Autodesk Inventor part; units mm, degrees
(part 6 of 6)
  arc A193 (71.9714, -302.9558) -> (71.5938, -302.4165) centre (71.5537, -302.8464) ccw
  arc A194 (71.5938, -302.4165) -> (70.7191, -302.3472) centre (68.6893, -333.536) ccw
  arc A195 (70.7191, -302.3472) -> (70.2313, -302.8189) centre (70.6894, -302.8046) ccw
  arc A196 (68.6893, -304.4648) -> (70.2313, -302.8189) centre (68.6351, -302.8687) ccw
  arc A197 (67.1472, -302.8189) -> (68.6893, -304.4648) centre (68.6385, -302.9671) ccw
  arc A198 (67.1472, -302.8189) -> (66.6899, -302.3453) centre (66.7175, -302.7762) ccw
  arc A199 (66.6899, -302.3453) -> (65.8152, -302.4137) centre (68.6893, -333.536) ccw
  circle A200 centre (68.6893, -333.536) radius 14.1111
  circle A201 centre (73.3883, -316.503) radius 2.0193
  circle A202 centre (51.5888, -337.983) radius 2.0193
  circle A203 centre (85.7897, -329.089) radius 2.0193
  circle A204 centre (56.2878, -320.95) radius 2.0193
  circle A205 centre (63.9903, -350.5689) radius 2.0193
  circle A206 centre (81.0907, -346.1219) radius 2.0193
  line L0 (-99.6407, 85.3463) -> (-99.6407, -123.6777) projected
  line L1 (-99.6407, -123.6777) -> (-99.6407, -461.902)
  arc A207 (-67.782, -300.7465) -> (-68.1901, -301.2886) centre (-67.7399, -301.2029) ccw
  arc A208 (-69.4556, -303.1555) -> (-68.1901, -301.2886) centre (-69.7588, -301.5876) ccw
  arc A209 (-71.2362, -301.7711) -> (-69.4556, -303.1555) centre (-69.7401, -301.6842) ccw
  arc A210 (-71.2362, -301.7711) -> (-71.762, -301.3749) centre (-71.6673, -301.7962) ccw
  arc A211 (-71.762, -301.3749) -> (-72.6152, -301.5793) centre (-64.9079, -331.8688) ccw
  arc A212 (-72.6152, -301.5793) -> (-72.9334, -302.1786) centre (-72.5022, -302.0234) ccw
  arc A213 (-73.8914, -304.2205) -> (-72.9334, -302.1786) centre (-74.4361, -302.7192) ccw
  arc A214 (-75.8666, -303.1316) -> (-73.8914, -304.2205) centre (-74.4025, -302.8117) ccw
  arc A215 (-75.8666, -303.1316) -> (-76.4479, -302.8225) centre (-76.2884, -303.2238) ccw
  arc A216 (-76.4479, -302.8225) -> (-77.2586, -303.1579) centre (-64.9079, -331.8688) ccw
  arc A217 (-77.2586, -303.1579) -> (-77.4792, -303.7996) centre (-77.0775, -303.5789) ccw
  arc A218 (-78.1059, -305.9662) -> (-77.4792, -303.7996) centre (-78.8788, -304.5687) ccw
  arc A219 (-80.2272, -305.1997) -> (-78.1059, -305.9662) centre (-78.8312, -304.6547) ccw
  arc A220 (-80.2272, -305.1997) -> (-80.8496, -304.9854) centre (-80.6294, -305.3568) ccw
  arc A221 (-80.8496, -304.9854) -> (-81.598, -305.4434) centre (-64.9079, -331.8688) ccw
  arc A222 (-81.598, -305.4434) -> (-81.7154, -306.1117) centre (-81.3532, -305.8309) ccw
  arc A223 (-81.9955, -308.3497) -> (-81.7154, -306.1117) centre (-82.9774, -307.0903) ccw
  arc A224 (-84.2105, -307.9245) -> (-81.9955, -308.3497) centre (-82.917, -307.1679) ccw
  arc A225 (-84.2105, -307.9245) -> (-84.8589, -307.8102) centre (-84.5832, -308.1426) ccw
  arc A226 (-84.8589, -307.8102) -> (-85.5263, -308.3797) centre (-64.9079, -331.8688) ccw
  arc A227 (-85.5263, -308.3797) -> (-85.5378, -309.0581) centre (-85.224, -308.7241) ccw
  arc A228 (-85.4643, -311.3124) -> (-85.5378, -309.0581) centre (-86.6312, -310.2221) ccw
  arc A229 (-87.7186, -311.2389) -> (-85.4643, -311.3124) centre (-86.5593, -310.2892) ccw
  arc A230 (-87.7186, -311.2389) -> (-88.3768, -311.2274) centre (-88.0526, -311.5126) ccw
  arc A231 (-88.3768, -311.2274) -> (-88.947, -311.8943) centre (-64.9079, -331.8688) ccw
  arc A232 (-88.947, -311.8943) -> (-88.8522, -312.5662) centre (-88.5945, -312.1872) ccw
  arc A233 (-88.427, -314.7812) -> (-88.8522, -312.5662) centre (-89.75, -313.8868) ccw
  arc A234 (-90.6649, -315.0613) -> (-88.427, -314.7812) centre (-89.6685, -313.9419) ccw
  arc A235 (-90.6649, -315.0613) -> (-91.3169, -315.1529) centre (-90.9521, -315.3838) ccw
  arc A236 (-91.3169, -315.1529) -> (-91.7757, -315.9007) centre (-64.9079, -331.8688) ccw
  arc A237 (-91.7757, -315.9007) -> (-91.577, -316.5495) centre (-91.3817, -316.1349) ccw
  arc A238 (-90.8105, -318.6707) -> (-91.577, -316.5495) centre (-92.2572, -317.9944) ccw
  arc A239 (-92.9771, -319.2975) -> (-90.8105, -318.6707) centre (-92.1681, -318.036) ccw
  arc A240 (-92.9771, -319.2975) -> (-93.6067, -319.4899) centre (-93.2102, -319.661) ccw
  arc A241 (-93.6067, -319.4899) -> (-93.9429, -320.3004) centre (-64.9079, -331.8688) ccw
  arc A242 (-93.9429, -320.3004) -> (-93.6451, -320.9101) centre (-93.5171, -320.47) ccw
  arc A243 (-92.5562, -322.8853) -> (-93.6451, -320.9101) centre (-94.0909, -322.4436) ccw
  arc A244 (-94.5981, -323.8433) -> (-92.5562, -322.8853) centre (-93.9964, -322.4708) ccw
  arc A245 (-94.5981, -323.8433) -> (-95.1899, -324.1318) centre (-94.7715, -324.2387) ccw
  arc A246 (-95.1899, -324.1318) -> (-95.3951, -324.9849) centre (-64.9079, -331.8688) ccw
  arc A247 (-95.3951, -324.9849) -> (-95.0056, -325.5405) centre (-94.9481, -325.0858) ccw
  arc A248 (-93.6212, -327.321) -> (-95.0056, -325.5405) centre (-95.206, -327.1248) ccw
  arc A249 (-95.488, -328.5866) -> (-93.6212, -327.321) centre (-95.1084, -327.1369) ccw
  arc A250 (-95.488, -328.5866) -> (-96.0274, -328.9642) centre (-95.5974, -329.0043) ccw
  arc A251 (-96.0274, -328.9642) -> (-96.0966, -329.8389) centre (-64.9079, -331.8688) ccw
  arc A252 (-96.0966, -329.8389) -> (-95.625, -330.3267) centre (-95.6393, -329.8686) ccw
  arc A253 (-93.9791, -331.8688) -> (-95.625, -330.3267) centre (-95.5751, -331.9229) ccw
  arc A254 (-95.625, -333.4108) -> (-93.9791, -331.8688) centre (-95.4768, -331.9196) ccw
  arc A255 (-95.625, -333.4108) -> (-96.0986, -333.8681) centre (-95.6677, -333.8405) ccw
  arc A256 (-96.0986, -333.8681) -> (-96.0302, -334.7429) centre (-64.9079, -331.8688) ccw
  arc A257 (-96.0302, -334.7429) -> (-95.488, -335.1509) centre (-95.5738, -334.7007) ccw
  arc A258 (-93.6212, -336.4165) -> (-95.488, -335.1509) centre (-95.1891, -336.7196) ccw
  arc A259 (-95.0056, -338.1971) -> (-93.6212, -336.4165) centre (-95.0925, -336.701) ccw
  arc A260 (-95.0056, -338.1971) -> (-95.4018, -338.7228) centre (-94.9805, -338.6281) ccw
  arc A261 (-95.4018, -338.7228) -> (-95.1974, -339.5761) centre (-64.9079, -331.8688) ccw
  arc A262 (-95.1974, -339.5761) -> (-94.5981, -339.8943) centre (-94.7533, -339.4631) ccw
  arc A263 (-92.5562, -340.8523) -> (-94.5981, -339.8943) centre (-94.0574, -341.3969) ccw
  arc A264 (-93.6451, -342.8275) -> (-92.5562, -340.8523) centre (-93.965, -341.3634) ccw
  arc A265 (-93.6451, -342.8275) -> (-93.9542, -343.4087) centre (-93.5529, -343.2493) ccw
  arc A266 (-93.9542, -343.4087) -> (-93.6188, -344.2195) centre (-64.9079, -331.8688) ccw
  arc A267 (-93.6188, -344.2195) -> (-92.9771, -344.44) centre (-93.1978, -344.0384) ccw
  arc A268 (-90.8105, -345.0668) -> (-92.9771, -344.44) centre (-92.208, -345.8396) ccw
  arc A269 (-91.577, -347.188) -> (-90.8105, -345.0668) centre (-92.1219, -345.792) ccw
  arc A270 (-91.577, -347.188) -> (-91.7913, -347.8105) centre (-91.4199, -347.5902) ccw
  arc A271 (-91.7913, -347.8105) -> (-91.3333, -348.5588) centre (-64.9079, -331.8688) ccw
  arc A272 (-91.3333, -348.5588) -> (-90.6649, -348.6763) centre (-90.9458, -348.3141) ccw
  arc A273 (-88.427, -348.9564) -> (-90.6649, -348.6763) centre (-89.6864, -349.9383) ccw
  arc A274 (-88.8522, -351.1714) -> (-88.427, -348.9564) centre (-89.6088, -349.8778) ccw
  arc A275 (-88.8522, -351.1714) -> (-88.9665, -351.8197) centre (-88.6341, -351.5441) ccw
  arc A276 (-88.9665, -351.8197) -> (-88.397, -352.4872) centre (-64.9079, -331.8688) ccw
  arc A277 (-88.397, -352.4872) -> (-87.7186, -352.4986) centre (-88.0526, -352.1848) ccw
  arc A278 (-85.4643, -352.4252) -> (-87.7186, -352.4986) centre (-86.5546, -353.592) ccw
  arc A279 (-85.5378, -354.6794) -> (-85.4643, -352.4252) centre (-86.4875, -353.5202) ccw
  arc A280 (-85.5378, -354.6794) -> (-85.5493, -355.3377) centre (-85.2641, -355.0134) ccw
  arc A281 (-85.5493, -355.3377) -> (-84.8824, -355.9078) centre (-64.9079, -331.8688) ccw
  arc A282 (-84.8824, -355.9078) -> (-84.2105, -355.813) centre (-84.5895, -355.5553) ccw
  arc A283 (-81.9955, -355.3878) -> (-84.2105, -355.813) centre (-82.8899, -356.7109) ccw
  arc A284 (-81.7154, -357.6258) -> (-81.9955, -355.3878) centre (-82.8348, -356.6294) ccw
  arc A285 (-81.7154, -357.6258) -> (-81.6238, -358.2778) centre (-81.3929, -357.9129) ccw
  arc A286 (-81.6238, -358.2778) -> (-80.8759, -358.7366) centre (-64.9079, -331.8688) ccw
  arc A287 (-80.8759, -358.7366) -> (-80.2272, -358.5378) centre (-80.6418, -358.3426) ccw
  arc A288 (-78.1059, -357.7714) -> (-80.2272, -358.5378) centre (-78.7823, -359.218) ccw
  arc A289 (-77.4792, -359.938) -> (-78.1059, -357.7714) centre (-78.7406, -359.1289) ccw
  arc A290 (-77.4792, -359.938) -> (-77.2867, -360.5676) centre (-77.1157, -360.1711) ccw
  arc A291 (-77.2867, -360.5676) -> (-76.4763, -360.9037) centre (-64.9079, -331.8688) ccw
  arc A292 (-76.4763, -360.9037) -> (-75.8666, -360.6059) centre (-76.3067, -360.478) ccw
  arc A293 (-73.8914, -359.5171) -> (-75.8666, -360.6059) centre (-74.3331, -361.0518) ccw
  arc A294 (-72.9334, -361.559) -> (-73.8914, -359.5171) centre (-74.3059, -360.9572) ccw
  arc A295 (-72.9334, -361.559) -> (-72.6449, -362.1507) centre (-72.538, -361.7324) ccw
  arc A296 (-72.6449, -362.1507) -> (-71.7918, -362.356) centre (-64.9079, -331.8688) ccw
  arc A297 (-71.7918, -362.356) -> (-71.2362, -361.9664) centre (-71.6909, -361.9089) ccw
  arc A298 (-69.4556, -360.582) -> (-71.2362, -361.9664) centre (-69.6519, -362.1669) ccw
  arc A299 (-68.1901, -362.4489) -> (-69.4556, -360.582) centre (-69.6398, -362.0693) ccw
  arc A300 (-68.1901, -362.4489) -> (-67.8125, -362.9882) centre (-67.7723, -362.5583) ccw
  arc A301 (-67.8125, -362.9882) -> (-66.9378, -363.0575) centre (-64.9079, -331.8688) ccw
  arc A302 (-66.9378, -363.0575) -> (-66.45, -362.5858) centre (-66.908, -362.6002) ccw
  arc A303 (-64.9079, -360.9399) -> (-66.45, -362.5858) centre (-64.8538, -362.536) ccw
  arc A304 (-63.3659, -362.5858) -> (-64.9079, -360.9399) centre (-64.8571, -362.4377) ccw
  arc A305 (-63.3659, -362.5858) -> (-62.9086, -363.0595) centre (-62.9362, -362.6285) ccw
  arc A306 (-62.9086, -363.0595) -> (-62.0338, -362.991) centre (-64.9079, -331.8688) ccw
  arc A307 (-62.0338, -362.991) -> (-61.6258, -362.4489) centre (-62.076, -362.5347) ccw
  arc A308 (-60.3602, -360.582) -> (-61.6258, -362.4489) centre (-60.057, -362.15) ccw
  arc A309 (-58.5796, -361.9664) -> (-60.3602, -360.582) centre (-60.0757, -362.0534) ccw
  arc A310 (-58.5796, -361.9664) -> (-58.0539, -362.3627) centre (-58.1486, -361.9414) ccw
  arc A311 (-58.0539, -362.3627) -> (-57.2006, -362.1583) centre (-64.9079, -331.8688) ccw
  arc A312 (-57.2006, -362.1583) -> (-56.8824, -361.559) centre (-57.3136, -361.7141) ccw
  arc A313 (-55.9244, -359.5171) -> (-56.8824, -361.559) centre (-55.3797, -361.0183) ccw
  arc A314 (-53.9492, -360.6059) -> (-55.9244, -359.5171) centre (-55.4133, -360.9258) ccw
  arc A315 (-53.9492, -360.6059) -> (-53.368, -360.915) centre (-53.5274, -360.5137) ccw
  arc A316 (-53.368, -360.915) -> (-52.5572, -360.5797) centre (-64.9079, -331.8688) ccw
  arc A317 (-52.5572, -360.5797) -> (-52.3366, -359.938) centre (-52.7383, -360.1587) ccw
  arc A318 (-51.7099, -357.7714) -> (-52.3366, -359.938) centre (-50.9371, -359.1689) ccw
  arc A319 (-49.5887, -358.5378) -> (-51.7099, -357.7714) centre (-50.9847, -359.0828) ccw
  arc A320 (-49.5887, -358.5378) -> (-48.9662, -358.7522) centre (-49.1864, -358.3808) ccw
  arc A321 (-48.9662, -358.7522) -> (-48.2179, -358.2941) centre (-64.9079, -331.8688) ccw
  arc A322 (-48.2179, -358.2941) -> (-48.1004, -357.6258) centre (-48.4626, -357.9066) ccw
  arc A323 (-47.8203, -355.3878) -> (-48.1004, -357.6258) centre (-46.8384, -356.6472) ccw
  arc A324 (-45.6053, -355.813) -> (-47.8203, -355.3878) centre (-46.8989, -356.5697) ccw
  arc A325 (-45.6053, -355.813) -> (-44.957, -355.9274) centre (-45.2326, -355.595) ccw
  arc A326 (-44.957, -355.9274) -> (-44.2895, -355.3579) centre (-64.9079, -331.8688) ccw
  arc A327 (-44.2895, -355.3579) -> (-44.2781, -354.6794) centre (-44.5919, -355.0134) ccw
  arc A328 (-44.3515, -352.4252) -> (-44.2781, -354.6794) centre (-43.1846, -353.5155) ccw
  arc A329 (-42.0973, -352.4986) -> (-44.3515, -352.4252) centre (-43.2565, -353.4483) ccw
  arc A330 (-42.0973, -352.4986) -> (-41.439, -352.5102) centre (-41.7632, -352.225) ccw
  arc A331 (-41.439, -352.5102) -> (-40.8689, -351.8433) centre (-64.9079, -331.8688) ccw
  arc A332 (-40.8689, -351.8433) -> (-40.9637, -351.1714) centre (-41.2214, -351.5504) ccw
  arc A333 (-41.3889, -348.9564) -> (-40.9637, -351.1714) centre (-40.0658, -349.8507) ccw
  arc A334 (-39.1509, -348.6763) -> (-41.3889, -348.9564) centre (-40.1473, -349.7956) ccw
  arc A335 (-39.1509, -348.6763) -> (-38.4989, -348.5847) centre (-38.8638, -348.3537) ccw
  arc A336 (-38.4989, -348.5847) -> (-38.0401, -347.8368) centre (-64.9079, -331.8688) ccw
  arc A337 (-38.0401, -347.8368) -> (-38.2389, -347.188) centre (-38.4341, -347.6027) ccw
  arc A338 (-39.0053, -345.0668) -> (-38.2389, -347.188) centre (-37.5587, -345.7432) ccw
  arc A339 (-36.8387, -344.44) -> (-39.0053, -345.0668) centre (-37.6478, -345.7015) ccw
  arc A340 (-36.8387, -344.44) -> (-36.2091, -344.2476) centre (-36.6056, -344.0766) ccw
  arc A341 (-36.2091, -344.2476) -> (-35.873, -343.4372) centre (-64.9079, -331.8688) ccw
  arc A342 (-35.873, -343.4372) -> (-36.1708, -342.8275) centre (-36.2987, -343.2675) ccw
  arc A343 (-37.2596, -340.8523) -> (-36.1708, -342.8275) centre (-35.7249, -341.294) ccw
  arc A344 (-35.2177, -339.8943) -> (-37.2596, -340.8523) centre (-35.8195, -341.2668) ccw
  arc A345 (-35.2177, -339.8943) -> (-34.626, -339.6057) centre (-35.0443, -339.4988) ccw
  arc A346 (-34.626, -339.6057) -> (-34.4207, -338.7527) centre (-64.9079, -331.8688) ccw
  arc A347 (-34.4207, -338.7527) -> (-34.8103, -338.1971) centre (-34.8678, -338.6517) ccw
  arc A348 (-36.1947, -336.4165) -> (-34.8103, -338.1971) centre (-34.6098, -336.6127) ccw
  arc A349 (-34.3278, -335.1509) -> (-36.1947, -336.4165) centre (-34.7074, -336.6006) ccw
  arc A350 (-34.3278, -335.1509) -> (-33.7885, -334.7733) centre (-34.2184, -334.7332) ccw
  arc A351 (-33.7885, -334.7733) -> (-33.7192, -333.8987) centre (-64.9079, -331.8688) ccw
  arc A352 (-33.7192, -333.8987) -> (-34.1908, -333.4108) centre (-34.1765, -333.8689) ccw
  arc A353 (-35.8368, -331.8688) -> (-34.1908, -333.4108) centre (-34.2407, -331.8146) ccw
  arc A354 (-34.1908, -330.3267) -> (-35.8368, -331.8688) centre (-34.339, -331.818) ccw
  arc A355 (-34.1908, -330.3267) -> (-33.7172, -329.8694) centre (-34.1481, -329.897) ccw
  arc A356 (-33.7172, -329.8694) -> (-33.7856, -328.9947) centre (-64.9079, -331.8688) ccw
  arc A357 (-33.7856, -328.9947) -> (-34.3278, -328.5866) centre (-34.242, -329.0368) ccw
  arc A358 (-36.1947, -327.321) -> (-34.3278, -328.5866) centre (-34.6267, -327.0179) ccw
  arc A359 (-34.8103, -325.5405) -> (-36.1947, -327.321) centre (-34.7233, -327.0366) ccw
  arc A360 (-34.8103, -325.5405) -> (-34.414, -325.0147) centre (-34.8353, -325.1094) ccw
  arc A361 (-34.414, -325.0147) -> (-34.6184, -324.1615) centre (-64.9079, -331.8688) ccw
  arc A362 (-34.6184, -324.1615) -> (-35.2177, -323.8433) centre (-35.0626, -324.2745) ccw
  arc A363 (-37.2596, -322.8853) -> (-35.2177, -323.8433) centre (-35.7584, -322.3406) ccw
  arc A364 (-36.1708, -320.9101) -> (-37.2596, -322.8853) centre (-35.8509, -322.3741) ccw
  arc A365 (-36.1708, -320.9101) -> (-35.8616, -320.3288) centre (-36.2629, -320.4882) ccw
  arc A366 (-35.8616, -320.3288) -> (-36.197, -319.518) centre (-64.9079, -331.8688) ccw
  arc A367 (-36.197, -319.518) -> (-36.8387, -319.2975) centre (-36.618, -319.6991) ccw
  arc A368 (-39.0053, -318.6707) -> (-36.8387, -319.2975) centre (-37.6078, -317.8979) ccw
  arc A369 (-38.2389, -316.5495) -> (-39.0053, -318.6707) centre (-37.6939, -317.9455) ccw
  arc A370 (-38.2389, -316.5495) -> (-38.0245, -315.927) centre (-38.3959, -316.1473) ccw
  arc A371 (-38.0245, -315.927) -> (-38.4826, -315.1787) centre (-64.9079, -331.8688) ccw
  arc A372 (-38.4826, -315.1787) -> (-39.1509, -315.0613) centre (-38.8701, -315.4235) ccw
  arc A373 (-41.3889, -314.7812) -> (-39.1509, -315.0613) centre (-40.1294, -313.7992) ccw
  arc A374 (-40.9637, -312.5662) -> (-41.3889, -314.7812) centre (-40.207, -313.8597) ccw
  arc A375 (-40.9637, -312.5662) -> (-40.8493, -311.9178) centre (-41.1817, -312.1935) ccw
  arc A376 (-40.8493, -311.9178) -> (-41.4188, -311.2504) centre (-64.9079, -331.8688) ccw
  arc A377 (-41.4188, -311.2504) -> (-42.0973, -311.2389) centre (-41.7632, -311.5527) ccw
  arc A378 (-44.3515, -311.3124) -> (-42.0973, -311.2389) centre (-43.2612, -310.1455) ccw
  arc A379 (-44.2781, -309.0581) -> (-44.3515, -311.3124) centre (-43.3284, -310.2174) ccw
  arc A380 (-44.2781, -309.0581) -> (-44.2665, -308.3999) centre (-44.5517, -308.7241) ccw
  arc A381 (-44.2665, -308.3999) -> (-44.9334, -307.8297) centre (-64.9079, -331.8688) ccw
  arc A382 (-44.9334, -307.8297) -> (-45.6053, -307.9245) centre (-45.2263, -308.1822) ccw
  arc A383 (-47.8203, -308.3497) -> (-45.6053, -307.9245) centre (-46.926, -307.0267) ccw
  arc A384 (-48.1004, -306.1117) -> (-47.8203, -308.3497) centre (-46.9811, -307.1082) ccw
  arc A385 (-48.1004, -306.1117) -> (-48.192, -305.4598) centre (-48.4229, -305.8246) ccw
  arc A386 (-48.192, -305.4598) -> (-48.9399, -305.001) centre (-64.9079, -331.8688) ccw
  arc A387 (-48.9399, -305.001) -> (-49.5887, -305.1997) centre (-49.174, -305.3949) ccw
  arc A388 (-51.7099, -305.9662) -> (-49.5887, -305.1997) centre (-51.0335, -304.5195) ccw
  arc A389 (-52.3366, -303.7996) -> (-51.7099, -305.9662) centre (-51.0752, -304.6086) ccw
  arc A390 (-52.3366, -303.7996) -> (-52.5291, -303.17) centre (-52.7001, -303.5665) ccw
  arc A391 (-52.5291, -303.17) -> (-53.3395, -302.8338) centre (-64.9079, -331.8688) ccw
  arc A392 (-53.3395, -302.8338) -> (-53.9492, -303.1316) centre (-53.5092, -303.2596) ccw
  arc A393 (-55.9244, -304.2205) -> (-53.9492, -303.1316) centre (-55.4827, -302.6858) ccw
  arc A394 (-56.8824, -302.1786) -> (-55.9244, -304.2205) centre (-55.5099, -302.7803) ccw
  arc A395 (-56.8824, -302.1786) -> (-57.171, -301.5868) centre (-57.2779, -302.0052) ccw
  arc A396 (-57.171, -301.5868) -> (-58.024, -301.3816) centre (-64.9079, -331.8688) ccw
  arc A397 (-58.024, -301.3816) -> (-58.5796, -301.7711) centre (-58.125, -301.8286) ccw
  arc A398 (-60.3602, -303.1555) -> (-58.5796, -301.7711) centre (-60.164, -301.5707) ccw
  arc A399 (-61.6258, -301.2886) -> (-60.3602, -303.1555) centre (-60.1761, -301.6683) ccw
  arc A400 (-61.6258, -301.2886) -> (-62.0034, -300.7493) centre (-62.0435, -301.1793) ccw
  arc A401 (-62.0034, -300.7493) -> (-62.878, -300.6801) centre (-64.9079, -331.8688) ccw
  arc A402 (-62.878, -300.6801) -> (-63.3659, -301.1517) centre (-62.9078, -301.1374) ccw
  arc A403 (-64.9079, -302.7976) -> (-63.3659, -301.1517) centre (-64.9621, -301.2016) ccw
  arc A404 (-66.45, -301.1517) -> (-64.9079, -302.7976) centre (-64.9587, -301.2999) ccw
  arc A405 (-66.45, -301.1517) -> (-66.9073, -300.6781) centre (-66.8797, -301.109) ccw
  arc A406 (-66.9073, -300.6781) -> (-67.782, -300.7465) centre (-64.9079, -331.8688) ccw
  circle A407 centre (-64.9079, -331.8688) radius 14.1111
  circle A408 centre (-60.2089, -314.8359) radius 2.0193
  circle A409 centre (-82.0084, -336.3158) radius 2.0193
  circle A410 centre (-47.8075, -327.4218) radius 2.0193
  circle A411 centre (-77.3094, -319.2829) radius 2.0193
  circle A412 centre (-69.6069, -348.9017) radius 2.0193
  circle A413 centre (-52.5065, -344.4547) radius 2.0193
  arc A414 (-1.7986, -301.6927) -> (-2.2066, -302.2349) centre (-1.7564, -302.1491) ccw
  arc A415 (-3.4722, -304.1017) -> (-2.2066, -302.2349) centre (-3.7754, -302.5338) ccw
  arc A416 (-5.2528, -302.7173) -> (-3.4722, -304.1017) centre (-3.7567, -302.6304) ccw
  arc A417 (-5.2528, -302.7173) -> (-5.7785, -302.3211) centre (-5.6839, -302.7424) ccw
  arc A418 (-5.7785, -302.3211) -> (-6.6318, -302.5255) centre (1.0755, -332.815) ccw
  arc A419 (-6.6318, -302.5255) -> (-6.95, -303.1248) centre (-6.5188, -302.9696) ccw
  arc A420 (-7.908, -305.1667) -> (-6.95, -303.1248) centre (-8.4527, -303.6655) ccw
  arc A421 (-9.8832, -304.0778) -> (-7.908, -305.1667) centre (-8.4191, -303.7579) ccw
  arc A422 (-9.8832, -304.0778) -> (-10.4645, -303.7687) centre (-10.305, -304.17) ccw
  arc A423 (-10.4645, -303.7687) -> (-11.2752, -304.1041) centre (1.0755, -332.815) ccw
  arc A424 (-11.2752, -304.1041) -> (-11.4958, -304.7458) centre (-11.0941, -304.5251) ccw
  arc A425 (-12.1225, -306.9124) -> (-11.4958, -304.7458) centre (-12.8954, -305.5149) ccw
  arc A426 (-14.2437, -306.1459) -> (-12.1225, -306.9124) centre (-12.8478, -305.601) ccw
  arc A427 (-14.2437, -306.1459) -> (-14.8662, -305.9316) centre (-14.646, -306.303) ccw
  arc A428 (-14.8662, -305.9316) -> (-15.6145, -306.3896) centre (1.0755, -332.815) ccw
  arc A429 (-15.6145, -306.3896) -> (-15.732, -307.058) centre (-15.3698, -306.7771) ccw
  arc A430 (-16.0121, -309.2959) -> (-15.732, -307.058) centre (-16.994, -308.0365) ccw
  arc A431 (-18.2271, -308.8707) -> (-16.0121, -309.2959) centre (-16.9335, -308.1141) ccw
  arc A432 (-18.2271, -308.8707) -> (-18.8754, -308.7564) centre (-18.5998, -309.0888) ccw
  arc A433 (-18.8754, -308.7564) -> (-19.5429, -309.3259) centre (1.0755, -332.815) ccw
  arc A434 (-19.5429, -309.3259) -> (-19.5544, -310.0043) centre (-19.2406, -309.6703) ccw
  arc A435 (-19.4809, -312.2586) -> (-19.5544, -310.0043) centre (-20.6478, -311.1683) ccw
  arc A436 (-21.7351, -312.1851) -> (-19.4809, -312.2586) centre (-20.5759, -311.2354) ccw
  arc A437 (-21.7351, -312.1851) -> (-22.3934, -312.1736) centre (-22.0692, -312.4588) ccw
  arc A438 (-22.3934, -312.1736) -> (-22.9636, -312.8405) centre (1.0755, -332.815) ccw
  arc A439 (-22.9636, -312.8405) -> (-22.8687, -313.5124) centre (-22.6111, -313.1334) ccw
  arc A440 (-22.4436, -315.7274) -> (-22.8687, -313.5124) centre (-23.7666, -314.833) ccw
  arc A441 (-24.6815, -316.0075) -> (-22.4436, -315.7274) centre (-23.6851, -314.8881) ccw
  arc A442 (-24.6815, -316.0075) -> (-25.3335, -316.0991) centre (-24.9686, -316.33) ccw
  arc A443 (-25.3335, -316.0991) -> (-25.7923, -316.847) centre (1.0755, -332.815) ccw
  arc A444 (-25.7923, -316.847) -> (-25.5935, -317.4957) centre (-25.3983, -317.0811) ccw
  arc A445 (-24.8271, -319.617) -> (-25.5935, -317.4957) centre (-26.2738, -318.9406) ccw
  arc A446 (-26.9937, -320.2437) -> (-24.8271, -319.617) centre (-26.1846, -318.9823) ccw
  arc A447 (-26.9937, -320.2437) -> (-27.6233, -320.4362) centre (-27.2268, -320.6072) ccw
  arc A448 (-27.6233, -320.4362) -> (-27.9595, -321.2466) centre (1.0755, -332.815) ccw
  arc A449 (-27.9595, -321.2466) -> (-27.6616, -321.8563) centre (-27.5337, -321.4162) ccw
  arc A450 (-26.5728, -323.8315) -> (-27.6616, -321.8563) centre (-28.1075, -323.3898) ccw
  arc A451 (-28.6147, -324.7895) -> (-26.5728, -323.8315) centre (-28.0129, -323.417) ccw
  arc A452 (-28.6147, -324.7895) -> (-29.2064, -325.078) centre (-28.7881, -325.1849) ccw
  arc A453 (-29.2064, -325.078) -> (-29.4117, -325.9311) centre (1.0755, -332.815) ccw
  arc A454 (-29.4117, -325.9311) -> (-29.0222, -326.4867) centre (-28.9646, -326.032) ccw
  arc A455 (-27.6377, -328.2673) -> (-29.0222, -326.4867) centre (-29.2226, -328.071) ccw
  arc A456 (-29.5046, -329.5328) -> (-27.6377, -328.2673) centre (-29.125, -328.0831) ccw
  arc A457 (-29.5046, -329.5328) -> (-30.0439, -329.9104) centre (-29.614, -329.9506) ccw
  arc A458 (-30.0439, -329.9104) -> (-30.1132, -330.7851) centre (1.0755, -332.815) ccw
  arc A459 (-30.1132, -330.7851) -> (-29.6416, -331.2729) centre (-29.6559, -330.8149) ccw
  arc A460 (-27.9957, -332.815) -> (-29.6416, -331.2729) centre (-29.5917, -332.8691) ccw
  arc A461 (-29.6416, -334.357) -> (-27.9957, -332.815) centre (-29.4934, -332.8658) ccw
  arc A462 (-29.6416, -334.357) -> (-30.1152, -334.8143) centre (-29.6843, -334.7867) ccw
  arc A463 (-30.1152, -334.8143) -> (-30.0468, -335.6891) centre (1.0755, -332.815) ccw
  arc A464 (-30.0468, -335.6891) -> (-29.5046, -336.0971) centre (-29.5904, -335.6469) ccw
  arc A465 (-27.6377, -337.3627) -> (-29.5046, -336.0971) centre (-29.2057, -337.6659) ccw
  arc A466 (-29.0222, -339.1433) -> (-27.6377, -337.3627) centre (-29.1091, -337.6472) ccw
  arc A467 (-29.0222, -339.1433) -> (-29.4184, -339.669) centre (-28.9971, -339.5743) ccw
  arc A468 (-29.4184, -339.669) -> (-29.214, -340.5223) centre (1.0755, -332.815) ccw
  arc A469 (-29.214, -340.5223) -> (-28.6147, -340.8405) centre (-28.7699, -340.4093) ccw
  arc A470 (-26.5728, -341.7985) -> (-28.6147, -340.8405) centre (-28.074, -342.3432) ccw
  arc A471 (-27.6616, -343.7737) -> (-26.5728, -341.7985) centre (-27.9816, -342.3096) ccw
  arc A472 (-27.6616, -343.7737) -> (-27.9708, -344.3549) centre (-27.5695, -344.1955) ccw
  arc A473 (-27.9708, -344.3549) -> (-27.6354, -345.1657) centre (1.0755, -332.815) ccw
  arc A474 (-27.6354, -345.1657) -> (-26.9937, -345.3863) centre (-27.2144, -344.9846) ccw
  arc A475 (-24.8271, -346.013) -> (-26.9937, -345.3863) centre (-26.2246, -346.7858) ccw
  arc A476 (-25.5935, -348.1342) -> (-24.8271, -346.013) centre (-26.1385, -346.7382) ccw
  arc A477 (-25.5935, -348.1342) -> (-25.8079, -348.7567) centre (-25.4365, -348.5365) ccw
  arc A478 (-25.8079, -348.7567) -> (-25.3498, -349.505) centre (1.0755, -332.815) ccw
  arc A479 (-25.3498, -349.505) -> (-24.6815, -349.6225) centre (-24.9624, -349.2603) ccw
  arc A480 (-22.4436, -349.9026) -> (-24.6815, -349.6225) centre (-23.703, -350.8845) ccw
  arc A481 (-22.8687, -352.1176) -> (-22.4436, -349.9026) centre (-23.6254, -350.824) ccw
  arc A482 (-22.8687, -352.1176) -> (-22.9831, -352.7659) centre (-22.6507, -352.4903) ccw
  arc A483 (-22.9831, -352.7659) -> (-22.4136, -353.4334) centre (1.0755, -332.815) ccw
  arc A484 (-22.4136, -353.4334) -> (-21.7351, -353.4448) centre (-22.0692, -353.131) ccw
  arc A485 (-19.4809, -353.3714) -> (-21.7351, -353.4448) centre (-20.5712, -354.5383) ccw
  arc A486 (-19.5544, -355.6256) -> (-19.4809, -353.3714) centre (-20.5041, -354.4664) ccw
  arc A487 (-19.5544, -355.6256) -> (-19.5659, -356.2839) centre (-19.2807, -355.9597) ccw
  arc A488 (-19.5659, -356.2839) -> (-18.899, -356.854) centre (1.0755, -332.815) ccw
  arc A489 (-18.899, -356.854) -> (-18.2271, -356.7592) centre (-18.6061, -356.5016) ccw
  arc A490 (-16.0121, -356.334) -> (-18.2271, -356.7592) centre (-16.9064, -357.6571) ccw
  arc A491 (-15.732, -358.572) -> (-16.0121, -356.334) centre (-16.8513, -357.5756) ccw
  arc A492 (-15.732, -358.572) -> (-15.6404, -359.224) centre (-15.4095, -358.8591) ccw
  arc A493 (-15.6404, -359.224) -> (-14.8925, -359.6828) centre (1.0755, -332.815) ccw
  arc A494 (-14.8925, -359.6828) -> (-14.2437, -359.484) centre (-14.6584, -359.2888) ccw
  arc A495 (-12.1225, -358.7176) -> (-14.2437, -359.484) centre (-12.7989, -360.1642) ccw
  arc A496 (-11.4958, -360.8842) -> (-12.1225, -358.7176) centre (-12.7572, -360.0751) ccw
  arc A497 (-11.4958, -360.8842) -> (-11.3033, -361.5138) centre (-11.1323, -361.1173) ccw
  arc A498 (-11.3033, -361.5138) -> (-10.4929, -361.8499) centre (1.0755, -332.815) ccw
  arc A499 (-10.4929, -361.8499) -> (-9.8832, -361.5521) centre (-10.3233, -361.4242) ccw
  arc A500 (-7.908, -360.4633) -> (-9.8832, -361.5521) centre (-8.3497, -361.998) ccw
  arc A501 (-6.95, -362.5052) -> (-7.908, -360.4633) centre (-8.3225, -361.9034) ccw
  arc A502 (-6.95, -362.5052) -> (-6.6614, -363.0969) centre (-6.5546, -362.6786) ccw
  arc A503 (-6.6614, -363.0969) -> (-5.8084, -363.3022) centre (1.0755, -332.815) ccw
  arc A504 (-5.8084, -363.3022) -> (-5.2528, -362.9127) centre (-5.7074, -362.8551) ccw
  arc A505 (-3.4722, -361.5282) -> (-5.2528, -362.9127) centre (-3.6684, -363.1131) ccw
  arc A506 (-2.2066, -363.3951) -> (-3.4722, -361.5282) centre (-3.6564, -363.0155) ccw
  arc A507 (-2.2066, -363.3951) -> (-1.829, -363.9344) centre (-1.7889, -363.5045) ccw
  arc A508 (-1.829, -363.9344) -> (-0.9544, -364.0037) centre (1.0755, -332.815) ccw
  arc A509 (-0.9544, -364.0037) -> (-0.4666, -363.5321) centre (-0.9246, -363.5464) ccw
  arc A510 (1.0755, -361.8861) -> (-0.4666, -363.5321) centre (1.1296, -363.4822) ccw
  arc A511 (2.6176, -363.5321) -> (1.0755, -361.8861) centre (1.1263, -363.3839) ccw
  arc A512 (2.6176, -363.5321) -> (3.0749, -364.0057) centre (3.0472, -363.5748) ccw
  arc A513 (3.0749, -364.0057) -> (3.9496, -363.9373) centre (1.0755, -332.815) ccw
  arc A514 (3.9496, -363.9373) -> (4.3576, -363.3951) centre (3.9074, -363.4809) ccw
  arc A515 (5.6232, -361.5282) -> (4.3576, -363.3951) centre (5.9264, -363.0962) ccw
  arc A516 (7.4038, -362.9127) -> (5.6232, -361.5282) centre (5.9077, -362.9996) ccw
  arc A517 (7.4038, -362.9127) -> (7.9295, -363.3089) centre (7.8349, -362.8876) ccw
  arc A518 (7.9295, -363.3089) -> (8.7828, -363.1045) centre (1.0755, -332.815) ccw
  arc A519 (8.7828, -363.1045) -> (9.101, -362.5052) centre (8.6698, -362.6603) ccw
  arc A520 (10.059, -360.4633) -> (9.101, -362.5052) centre (10.6037, -361.9645) ccw
  arc A521 (12.0342, -361.5521) -> (10.059, -360.4633) centre (10.5701, -361.872) ccw
  arc A522 (12.0342, -361.5521) -> (12.6155, -361.8613) centre (12.456, -361.46) ccw
  arc A523 (12.6155, -361.8613) -> (13.4262, -361.5259) centre (1.0755, -332.815) ccw
  arc A524 (13.4262, -361.5259) -> (13.6468, -360.8842) centre (13.2451, -361.1049) ccw
  arc A525 (14.2735, -358.7176) -> (13.6468, -360.8842) centre (15.0464, -360.1151) ccw
  arc A526 (16.3947, -359.484) -> (14.2735, -358.7176) centre (14.9988, -360.029) ccw
  arc A527 (16.3947, -359.484) -> (17.0172, -359.6984) centre (16.797, -359.327) ccw
  arc A528 (17.0172, -359.6984) -> (17.7655, -359.2403) centre (1.0755, -332.815) ccw
  arc A529 (17.7655, -359.2403) -> (17.883, -358.572) centre (17.5208, -358.8528) ccw
  arc A530 (18.1631, -356.334) -> (17.883, -358.572) centre (19.145, -357.5935) ccw
  arc A531 (20.3781, -356.7592) -> (18.1631, -356.334) centre (19.0845, -357.5159) ccw
  arc A532 (20.3781, -356.7592) -> (21.0264, -356.8736) centre (20.7508, -356.5412) ccw
  arc A533 (21.0264, -356.8736) -> (21.6939, -356.3041) centre (1.0755, -332.815) ccw
  arc A534 (21.6939, -356.3041) -> (21.7054, -355.6256) centre (21.3916, -355.9597) ccw
  arc A535 (21.6319, -353.3714) -> (21.7054, -355.6256) centre (22.7988, -354.4617) ccw
  arc A536 (23.8862, -353.4448) -> (21.6319, -353.3714) centre (22.7269, -354.3945) ccw
  arc A537 (23.8862, -353.4448) -> (24.5444, -353.4564) centre (24.2202, -353.1712) ccw
  arc A538 (24.5444, -353.4564) -> (25.1146, -352.7895) centre (1.0755, -332.815) ccw
  arc A539 (25.1146, -352.7895) -> (25.0197, -352.1176) centre (24.7621, -352.4966) ccw
  arc A540 (24.5946, -349.9026) -> (25.0197, -352.1176) centre (25.9176, -350.7969) ccw
  arc A541 (26.8325, -349.6225) -> (24.5946, -349.9026) centre (25.8361, -350.7418) ccw
  arc A542 (26.8325, -349.6225) -> (27.4845, -349.5309) centre (27.1196, -349.3) ccw
  arc A543 (27.4845, -349.5309) -> (27.9433, -348.783) centre (1.0755, -332.815) ccw
  arc A544 (27.9433, -348.783) -> (27.7445, -348.1342) centre (27.5493, -348.5489) ccw
  arc A545 (26.9781, -346.013) -> (27.7445, -348.1342) centre (28.4248, -346.6894) ccw
  arc A546 (29.1447, -345.3863) -> (26.9781, -346.013) centre (28.3357, -346.6477) ccw
  arc A547 (29.1447, -345.3863) -> (29.7743, -345.1938) centre (29.3778, -345.0228) ccw
  arc A548 (29.7743, -345.1938) -> (30.1105, -344.3834) centre (1.0755, -332.815) ccw
  arc A549 (30.1105, -344.3834) -> (29.8127, -343.7737) centre (29.6847, -344.2137) ccw
  arc A550 (28.7238, -341.7985) -> (29.8127, -343.7737) centre (30.2585, -342.2402) ccw
  arc A551 (30.7657, -340.8405) -> (28.7238, -341.7985) centre (30.164, -342.213) ccw
  arc A552 (30.7657, -340.8405) -> (31.3574, -340.5519) centre (30.9391, -340.445) ccw
  arc A553 (31.3574, -340.5519) -> (31.5627, -339.6989) centre (1.0755, -332.815) ccw
  arc A554 (31.5627, -339.6989) -> (31.1732, -339.1433) centre (31.1156, -339.5979) ccw
  arc A555 (29.7887, -337.3627) -> (31.1732, -339.1433) centre (31.3736, -337.5589) ccw
  arc A556 (31.6556, -336.0971) -> (29.7887, -337.3627) centre (31.276, -337.5468) ccw
  arc A557 (31.6556, -336.0971) -> (32.1949, -335.7195) centre (31.765, -335.6794) ccw
  arc A558 (32.1949, -335.7195) -> (32.2642, -334.8449) centre (1.0755, -332.815) ccw
  arc A559 (32.2642, -334.8449) -> (31.7926, -334.357) centre (31.8069, -334.8151) ccw
  arc A560 (30.1467, -332.815) -> (31.7926, -334.357) centre (31.7427, -332.7609) ccw
  arc A561 (31.7926, -331.2729) -> (30.1467, -332.815) centre (31.6444, -332.7642) ccw
  arc A562 (31.7926, -331.2729) -> (32.2662, -330.8156) centre (31.8353, -330.8432) ccw
  arc A563 (32.2662, -330.8156) -> (32.1978, -329.9409) centre (1.0755, -332.815) ccw
  arc A564 (32.1978, -329.9409) -> (31.6556, -329.5328) centre (31.7414, -329.983) ccw
  arc A565 (29.7887, -328.2673) -> (31.6556, -329.5328) centre (31.3567, -327.9641) ccw
  arc A566 (31.1732, -326.4867) -> (29.7887, -328.2673) centre (31.2601, -327.9828) ccw
  arc A567 (31.1732, -326.4867) -> (31.5694, -325.9609) centre (31.1481, -326.0556) ccw
  arc A568 (31.5694, -325.9609) -> (31.365, -325.1077) centre (1.0755, -332.815) ccw
  arc A569 (31.365, -325.1077) -> (30.7657, -324.7895) centre (30.9209, -325.2207) ccw
  arc A570 (28.7238, -323.8315) -> (30.7657, -324.7895) centre (30.225, -323.2868) ccw
  arc A571 (29.8127, -321.8563) -> (28.7238, -323.8315) centre (30.1326, -323.3204) ccw
  arc A572 (29.8127, -321.8563) -> (30.1218, -321.275) centre (29.7205, -321.4345) ccw
  arc A573 (30.1218, -321.275) -> (29.7864, -320.4643) centre (1.0755, -332.815) ccw
  arc A574 (29.7864, -320.4643) -> (29.1447, -320.2437) centre (29.3654, -320.6454) ccw
  arc A575 (26.9781, -319.617) -> (29.1447, -320.2437) centre (28.3756, -318.8441) ccw
  arc A576 (27.7445, -317.4957) -> (26.9781, -319.617) centre (28.2895, -318.8917) ccw
  arc A577 (27.7445, -317.4957) -> (27.9589, -316.8733) centre (27.5875, -317.0935) ccw
  arc A578 (27.9589, -316.8733) -> (27.5008, -316.1249) centre (1.0755, -332.815) ccw
  arc A579 (27.5008, -316.1249) -> (26.8325, -316.0075) centre (27.1134, -316.3697) ccw
  arc A580 (24.5946, -315.7274) -> (26.8325, -316.0075) centre (25.854, -314.7455) ccw
  arc A581 (25.0197, -313.5124) -> (24.5946, -315.7274) centre (25.7764, -314.8059) ccw
  arc A582 (25.0197, -313.5124) -> (25.1341, -312.864) centre (24.8017, -313.1397) ccw
  arc A583 (25.1341, -312.864) -> (24.5646, -312.1966) centre (1.0755, -332.815) ccw
  arc A584 (24.5646, -312.1966) -> (23.8862, -312.1851) centre (24.2202, -312.4989) ccw
  arc A585 (21.6319, -312.2586) -> (23.8862, -312.1851) centre (22.7222, -311.0917) ccw
  arc A586 (21.7054, -310.0043) -> (21.6319, -312.2586) centre (22.6551, -311.1636) ccw
  arc A587 (21.7054, -310.0043) -> (21.7169, -309.3461) centre (21.4317, -309.6703) ccw
  arc A588 (21.7169, -309.3461) -> (21.05, -308.7759) centre (1.0755, -332.815) ccw
  arc A589 (21.05, -308.7759) -> (20.3781, -308.8707) centre (20.7571, -309.1284) ccw
  arc A590 (18.1631, -309.2959) -> (20.3781, -308.8707) centre (19.0574, -307.9729) ccw
  arc A591 (17.883, -307.058) -> (18.1631, -309.2959) centre (19.0024, -308.0544) ccw
  arc A592 (17.883, -307.058) -> (17.7914, -306.406) centre (17.5605, -306.7708) ccw
  arc A593 (17.7914, -306.406) -> (17.0435, -305.9472) centre (1.0755, -332.815) ccw
  arc A594 (17.0435, -305.9472) -> (16.3947, -306.1459) centre (16.8094, -306.3412) ccw
  arc A595 (14.2735, -306.9124) -> (16.3947, -306.1459) centre (14.9499, -305.4657) ccw
  arc A596 (13.6468, -304.7458) -> (14.2735, -306.9124) centre (14.9082, -305.5548) ccw
  arc A597 (13.6468, -304.7458) -> (13.4543, -304.1162) centre (13.2833, -304.5127) ccw
  arc A598 (13.4543, -304.1162) -> (12.6439, -303.78) centre (1.0755, -332.815) ccw
  arc A599 (12.6439, -303.78) -> (12.0342, -304.0778) centre (12.4743, -304.2058) ccw
  arc A600 (10.059, -305.1667) -> (12.0342, -304.0778) centre (10.5007, -303.632) ccw
  arc A601 (9.101, -303.1248) -> (10.059, -305.1667) centre (10.4735, -303.7265) ccw
  arc A602 (9.101, -303.1248) -> (8.8124, -302.533) centre (8.7056, -302.9514) ccw
  arc A603 (8.8124, -302.533) -> (7.9594, -302.3278) centre (1.0755, -332.815) ccw
  arc A604 (7.9594, -302.3278) -> (7.4038, -302.7173) centre (7.8585, -302.7748) ccw
  arc A605 (5.6232, -304.1017) -> (7.4038, -302.7173) centre (5.8194, -302.5169) ccw
  arc A606 (4.3576, -302.2349) -> (5.6232, -304.1017) centre (5.8074, -302.6145) ccw
  arc A607 (4.3576, -302.2349) -> (3.9801, -301.6955) centre (3.9399, -302.1255) ccw
  arc A608 (3.9801, -301.6955) -> (3.1054, -301.6263) centre (1.0755, -332.815) ccw
  arc A609 (3.1054, -301.6263) -> (2.6176, -302.0979) centre (3.0756, -302.0836) ccw
  arc A610 (1.0755, -303.7438) -> (2.6176, -302.0979) centre (1.0214, -302.1478) ccw
  arc A611 (-0.4666, -302.0979) -> (1.0755, -303.7438) centre (1.0247, -302.2461) ccw
  arc A612 (-0.4666, -302.0979) -> (-0.9239, -301.6243) centre (-0.8962, -302.0552) ccw
  arc A613 (-0.9239, -301.6243) -> (-1.7986, -301.6927) centre (1.0755, -332.815) ccw
  circle A614 centre (1.0755, -332.815) radius 14.1111
  circle A615 centre (5.7745, -315.7821) radius 2.0193
  circle A616 centre (-16.0249, -337.262) radius 2.0193
  circle A617 centre (18.1759, -328.368) radius 2.0193
  circle A618 centre (-11.3259, -320.2291) radius 2.0193
  circle A619 centre (-3.6235, -349.8479) radius 2.0193
  circle A620 centre (13.4769, -345.4009) radius 2.0193
  point P0 (0, 0)
  constraints: 1200 point on circle, 621 centre point, 2 end point, 1 vertical
body "Solid1"
body "Solid2"
